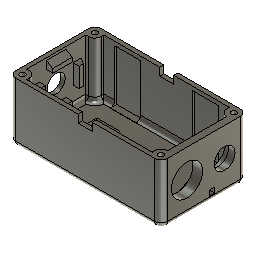
SolderungStationV2_Case_ESD_v2.8 (Autodesk Fusion 360 design; units mm, degrees)
Autodesk Fusion 360 part; units mm, degrees
sketch "草图1" plane through (0, 0, 0) normal (0, 0, 1) x (1, 0, 0)
  line L0 (2.5, 0) -> (56, 0)
  line L1 (58.5, -2.5) -> (58.5, -30.5)
  line L2 (56, -33) -> (2.5, -33)
  line L3 (0, -30.5) -> (0, -2.5)
  line L4 (0, -27.9) -> (2.6, -27.9)
  line L5 (5.1, -30.4) -> (5.1, -33)
  line L6 (58.5, -27.9) -> (55.9, -27.9)
  line L7 (53.4, -30.4) -> (53.4, -33)
  line L8 (53.4, 0) -> (53.4, -2.6)
  line L9 (55.9, -5.1) -> (58.5, -5.1)
  line L10 (5.1, 0) -> (5.1, -2.6)
  line L11 (2.6, -5.1) -> (0, -5.1)
  circle A0 centre (2.535, -2.53) radius 1
  line L12 (2.535, -2.53) -> (55.965, -2.53) construction
  line L13 (55.965, -2.53) -> (55.965, -30.47) construction
  line L14 (55.965, -30.47) -> (2.535, -30.47) construction
  line L15 (2.535, -30.47) -> (2.535, -2.53) construction
  circle A1 centre (55.965, -2.53) radius 1
  circle A2 centre (55.965, -30.47) radius 1
  circle A3 centre (2.535, -30.47) radius 1
  line L16 (2.535, -30.47) -> (0, -33) construction
  line L17 (55.965, -30.47) -> (58.5, -33) construction
  line L18 (58.5, 0) -> (55.965, -2.53) construction
  line L19 (0, 0) -> (2.535, -2.53) construction
  arc A4 (2.5, 0) -> (0, -2.5) centre (2.5, -2.5) ccw
  arc A5 (58.5, -2.5) -> (56, 0) centre (56, -2.5) ccw
  arc A6 (56, -33) -> (58.5, -30.5) centre (56, -30.5) ccw
  arc A7 (0, -30.5) -> (2.5, -33) centre (2.5, -30.5) ccw
  arc A8 (2.6, -5.1) -> (5.1, -2.6) centre (2.6, -2.6) ccw
  arc A9 (5.1, -30.4) -> (2.6, -27.9) centre (2.6, -30.4) ccw
  arc A10 (53.4, -2.6) -> (55.9, -5.1) centre (55.9, -2.6) ccw
  arc A11 (55.9, -27.9) -> (53.4, -30.4) centre (55.9, -30.4) ccw
  line L20 (56, -31.4) -> (2.5, -31.4)
  arc A12 (1.6, -30.5) -> (2.5, -31.4) centre (2.5, -30.5) ccw
  line L21 (1.6, -30.5) -> (1.6, -2.5)
  arc A13 (2.5, -1.6) -> (1.6, -2.5) centre (2.5, -2.5) ccw
  line L22 (2.5, -1.6) -> (56, -1.6)
  arc A14 (56.9, -2.5) -> (56, -1.6) centre (56, -2.5) ccw
  line L23 (56.9, -2.5) -> (56.9, -30.5)
  arc A15 (56, -31.4) -> (56.9, -30.5) centre (56, -30.5) ccw
  line L24 (55.96, -31.4) -> (55.96, -1.5)
  line L25 (10, -9.25) -> (18.9, -9.25)
  line L26 (18.9, -9.25) -> (18.9, -23.75)
  line L27 (18.9, -23.75) -> (10, -23.75)
  line L28 (10, -23.75) -> (10, -9.25)
  line L29 (0, -16.5) -> (58.5, -16.5)
  point P0 (5.1, -27.9)
  dimension "d1" = 58.5
  dimension "d2" = 33
  dimension "d5" = 1.6
  dimension "d6" = 5.1
  dimension "d7" = 2
  dimension "d10" = 53.43
  dimension "d11" = 27.94
  dimension "d12" = 2.5
  dimension "d28" = 2.5
  dimension "d37" = 2.54
  dimension "d75" = 14.5
  dimension "d77" = 8.9
  dimension "d78" = 10
  constraint horizontal L0
  constraint vertical L1
  constraint horizontal L2
  constraint vertical L3
  constraint coincident L19.start origin
  constraint coincident L3 L4.start
  constraint coincident L2 L5.end
  constraint perpendicular L2 L5
  constraint coincident L1 L6.start
  constraint perpendicular L1 L6
  constraint coincident L2 L7.end
  constraint perpendicular L2 L7
  constraint coincident L0 L8.start
  constraint perpendicular L0 L8
  constraint coincident L1 L9.end
  constraint perpendicular L1 L9
  constraint coincident L0 L10.start
  constraint perpendicular L10 L22
  constraint coincident L3 L11.end
  constraint perpendicular L3 L11
  constraint collinear L5 L10
  constraint collinear L4 L6
  constraint collinear L9 L11
  constraint horizontal L12
  constraint vertical L13
  constraint horizontal L14
  constraint vertical L15
  constraint coincident L12.end L13.start
  constraint coincident L13.end L14.start
  constraint coincident L14.end L15.start
  constraint coincident A0.centre L12.start
  constraint equal A0 A1
  constraint equal A0 A3
  constraint equal A0 A2
  constraint equal L16 L17
  constraint equal L17 L18
  constraint coincident L19.start L0
  constraint coincident L19.start L3
  constraint tangent L0 A4
  constraint tangent L3 A4
  constraint coincident L18.start L0
  constraint coincident L18.start L1
  constraint tangent L0 A5
  constraint tangent L1 A5
  constraint equal A4 A5
  constraint coincident L17.end L1
  constraint coincident L17.end L2
  constraint tangent L1 A6
  constraint tangent L2 A6
  constraint equal A4 A6
  constraint coincident L16.end L2
  constraint coincident L16.end L3
  constraint tangent L2 A7
  constraint tangent L3 A7
  constraint equal A4 A7
  constraint tangent L10 A8
  constraint tangent L11 A8
  constraint coincident P0 L5
  constraint coincident P0 L4
  constraint tangent L5 A9
  constraint tangent L4 A9
  constraint tangent L9 A10
  constraint tangent L8 A10
  constraint tangent L6 A11
  constraint tangent L7 A11
  constraint equal A9 A11
  constraint equal A8 A9
  constraint equal L4 L5
  constraint collinear L7 L8
  constraint equal A9 A10
  constraint equal L8 L9
  constraint equal L10 L11
  constraint coincident L20 L24.start
  constraint perpendicular L12 L24
  constraint horizontal L25
  constraint vertical L26
  constraint horizontal L27
  constraint vertical L28
  constraint midpoint L3 L29.start
  constraint midpoint L1 L29.end
  constraint symmetric L25 L27 L29
  measures "d1" distance of L19.start L18.start
  measures "d2" distance of L18.start L17.end
  measures "d6" distance of P0 L5.end
  measures "d7" diameter of A0
  measures "d10" distance of A0.centre L12.end
  measures "d11" distance of A0.centre L14.end
  measures "d12" radius of A4
  measures "d28" radius of A9
  measures "d37" distance of L1 L24
  measures "d75" distance of L25.end L26.end
  measures "d77" distance of L25.start L25.end
  measures "d78" distance of L3 L28
extrude "拉伸2" add sketch "草图1" along normal blind 1.6 contours L0 L3 L10 L11 A0 A4 L21 L22 | L0 L8 L10 L22 | L0 L1 L8 L9 A1 A5 L22 L23 | L8 L9 L10 L11 A8 A10 L21 L22 L24 L25 L26 L28 L29 | L10 L11 A0 A8 L21 L22 | L3 L11 L21 L29 | L8 L9 A1 A10 L22 L24 | A0 L21 A13 L22 | A0 L21 A13 L22 | L3 L4 L21 L29 | A1 L22 L24 | A1 L22 L24 | L2 L3 L4 L5 A3 A7 L20 L21 | L4 L5 L6 L7 A9 A11 L20 L21 L24 L26 L27 L28 L29 | L1 L9 L23 L29 | A1 L22 A14 L23 L24 | A1 L22 A14 L23 L24 | L9 A1 L23 L24 | L4 L5 A3 A9 L20 L21 | L1 L6 L23 L29 | L9 L23 L24 L29 | A3 L20 A12 L21 | A3 L20 A12 L21 | L1 L2 L6 L7 A2 A6 L20 L23 | L6 L23 L24 L29 | L2 L5 L7 L20 | L6 A2 L23 L24 | L6 L7 A2 A11 L20 L24 | A2 L20 L23 A15 L24 | A2 L20 L23 A15 | A2 L20 L24 makes body 1
extrude "拉伸3" add sketch "草图1" along normal blind 23 separate body contours L0 L3 L10 L11 A0 A4 L21 L22 | L0 L8 L10 L22 | L0 L1 L8 L9 A1 A5 L22 L23 | L10 L11 A0 A8 L21 L22 | L3 L11 L21 L29 | L8 L9 A1 A10 L22 L24 | A0 L21 A13 L22 | A0 L21 A13 L22 | L3 L4 L21 L29 | A1 L22 L24 | A1 L22 L24 | L2 L3 L4 L5 A3 A7 L20 L21 | L1 L9 L23 L29 | A1 L22 A14 L23 L24 | A1 L22 A14 L23 L24 | L9 A1 L23 L24 | L4 L5 A3 A9 L20 L21 | L1 L6 L23 L29 | L9 L23 L24 L29 | A3 L20 A12 L21 | A3 L20 A12 L21 | L1 L2 L6 L7 A2 A6 L20 L23 | L6 L23 L24 L29 | L2 L5 L7 L20 | L6 A2 L23 L24 | L6 L7 A2 A11 L20 L24 | A2 L20 L23 A15 L24 | A2 L20 L23 A15 | A2 L20 L24 makes body 2
combine "合并1" operation add target body 2 tool bodies 1
sketch "草图3" plane through (55.96, 0, 0) normal (-1, 0, 0) x (0, 1, 0)
  circle A0 centre (-23, -12) radius 6
  circle A1 centre (-8.5, -12) radius 4
  line L0 (-23, -12) -> (-8.5, -12) construction
  line L1 (-16.5, -1.6) -> (-16.5, -23) construction
  line L2 (-30.5, -16.3301) -> (-23, -20.6603)
  line L3 (-23, -20.6603) -> (-15.5, -16.3301)
  line L4 (-15.5, -16.3301) -> (-15.5, -7.6699)
  line L5 (-15.5, -7.6699) -> (-23, -3.3397)
  line L6 (-23, -3.3397) -> (-30.5, -7.6699)
  line L7 (-30.5, -7.6699) -> (-30.5, -16.3301)
  line L8 (-5.1, -1.6) -> (-27.9, -1.6)
  line L9 (-27.9, -1.6) -> (-27.9, -23)
  line L10 (-27.9, -23) -> (-5.1, -23)
  line L11 (-5.1, -23) -> (-5.1, -1.6)
  line L12 (-1, -12) -> (-32, -12)
  line L13 (-32, -12) -> (-32, -0.6011)
  line L14 (-32, -0.6011) -> (-1, -0.6011)
  line L15 (-1, -0.6011) -> (-1, -12)
  line L16 (-15.5, -16.3301) -> (-13.1332, -14.9637)
  line L17 (-13.5746, -14.121) -> (-13.5746, -15.2185)
  circle A2 centre (-8.5, -12) radius 5.5
  line L18 (-14.4011, -4.3276) -> (-12.4011, -4.3276)
  line L19 (-12.4011, -4.3276) -> (-12.4011, -2.3276)
  line L20 (-12.4011, -2.3276) -> (-14.4011, -2.3276)
  line L21 (-14.4011, -2.3276) -> (-14.4011, -4.3276)
  point P0 (-23, -12)
  point P1 (-8.5, -12)
  dimension "d31" = 12
  dimension "d32" = 8
  dimension "d34" = 6.5
  dimension "d35" = 8
  dimension "d38" = 7.5
  dimension "d39" = 11
  dimension "d51" = 11
  dimension "d99" = 2
  constraint coincident P0 A0.centre
  constraint coincident P1 A1.centre
  constraint horizontal L0
  constraint vertical L1
  constraint midpoint L1.end L10
  constraint midpoint L1.start L8
  constraint vertical L7
  constraint horizontal L12
  constraint vertical L13
  constraint horizontal L14
  constraint vertical L15
  constraint collinear L3 L16
  constraint coincident L16 L17.end
  constraint concentric A1 A2
  constraint coincident L16.end A2
  constraint collinear L0 L12
  constraint coincident L17.start A2
  constraint vertical L17
  constraint horizontal L18
  constraint vertical L19
  constraint horizontal L20
  constraint vertical L21
  constraint equal L18 L19
  measures "d31" diameter of A0
  measures "d32" diameter of A1
  measures "d34" distance of P0 L1
  measures "d35" distance of P1 L1
  measures "d38" distance of P0 L7
  measures "d39" distance of L0 L10
  measures "d51" diameter of A2
  measures "d99" distance of L18.start L18.end
extrude "拉伸7" add sketch "草图3" along normal blind 2.56 contours L4 L12 L16 L17 A2 | L4 L5 L6 L8 L9 L11 L12 A2 | L6 L7 L8 L9 L11 L12 L13 L14 L15 A2 | L18 L19 L20 L21 bodies 2
extrude "拉伸5" cut sketch "草图3" along normal blind 10 contours A0 L9 L12 | A0 L2 L3 L4 L9 L12 | A0 L4 L5 L6 L9 L12 | A0 L9 L12 | A0 L9 L12 | A0 L6 L7 L9 L12 | A0 L2 L7 L9 L12 | A0 L9 L12 | A1 L11 L12 A2 | A1 L11 L12 A2 | A1 L11 L12 | A1 L11 L12 | A1 L11 L12 A2 | A1 L11 L12 | A1 L11 L12 | A1 L11 L12 A2 bodies 2
extrude "拉伸8" add sketch "草图3" along normal blind 1.2 contours A0 L9 L12 | A0 L2 L3 L4 L9 L12 | A0 L4 L5 L6 L9 L12 | A0 L9 L12 | A0 L9 L12 | A0 L6 L7 L9 L12 | A0 L2 L7 L9 L12 | A0 L9 L12 bodies 2
extrude "拉伸4" cut sketch "草图3" along normal mid plane 10 contours A0 L9 L12 | A0 L9 L12 | A0 L9 L12 | A0 L9 L12 | A1 L11 L12 | A1 L11 L12 | A1 L11 L12 | A1 L11 L12 | L18 L19 L20 L21 bodies 2
sketch "草图2" plane through (0, 0, 23) normal (0, 0, 1) x (-1, 0, 0)
  line L0 (-5.1, 1.6) -> (-53.4, 1.6)
  line L1 (-53.4, 31.4) -> (-5.1, 31.4)
  line L2 (-1.6, 27.9) -> (-1.6, 5.1)
  arc A0 (-2.5, 0) -> (0, 2.5) centre (-2.5, 2.5) ccw
  line L3 (0, 2.5) -> (0, 30.5)
  arc A1 (0, 30.5) -> (-2.5, 33) centre (-2.5, 30.5) ccw
  line L4 (-2.5, 33) -> (-56, 33)
  arc A2 (-56, 33) -> (-58.5, 30.5) centre (-56, 30.5) ccw
  line L5 (-58.5, 30.5) -> (-58.5, 2.5)
  arc A3 (-58.5, 2.5) -> (-56, 0) centre (-56, 2.5) ccw
  line L6 (-56, 0) -> (-2.5, 0)
  circle A4 centre (-2.535, 30.47) radius 1
  circle A5 centre (-2.535, 2.53) radius 1
  circle A6 centre (-55.965, 2.53) radius 1
  circle A7 centre (-55.965, 30.47) radius 1
  line L7 (-5.1, 2.6) -> (-5.1, 1.6)
  line L8 (-53.4, 30.4) -> (-53.4, 31.4)
  arc A8 (-53.4, 2.6) -> (-55.9, 5.1) centre (-55.9, 2.6) ccw
  line L9 (-55.9, 5.1) -> (-55.96, 5.1)
  line L10 (-55.96, 27.9) -> (-55.9, 27.9)
  arc A9 (-55.9, 27.9) -> (-53.4, 30.4) centre (-55.9, 30.4) ccw
  line L11 (-5.1, 31.4) -> (-5.1, 30.4)
  arc A10 (-5.1, 30.4) -> (-2.6, 27.9) centre (-2.6, 30.4) ccw
  line L12 (-2.6, 27.9) -> (-1.6, 27.9)
  line L13 (-1.6, 5.1) -> (-2.6, 5.1)
  arc A11 (-2.6, 5.1) -> (-5.1, 2.6) centre (-2.6, 2.6) ccw
  line L14 (-53.4, 1.6) -> (-53.4, 2.6)
  line L15 (-55.96, 5.1) -> (-55.96, 27.9)
hole "孔1" at (2.535, -30.47, 23) at (2.535, -2.53, 23) at (56, -30.5, 23) at (56, -2.5, 23) direction (0, 0, -1) diameter 2 depth 8 tip angle 180 bodies 2
sketch "草图4" plane through (0, 0, 0) normal (0, 1, 0) x (1, 0, 0)
  line L0 (2.5, 0) -> (2.5, -23)
  line L1 (2.5, -23) -> (56, -23)
  line L2 (56, -23) -> (56, 0)
  line L3 (56, 0) -> (2.5, 0)
  line L4 (0, 0) -> (0, -23)
  line L5 (0, -23) -> (2.5, -23)
  line L6 (2.5, -23) -> (2.5, 0)
  line L7 (0, 0) -> (2.5, 0)
  line L8 (56, 0) -> (56, -23)
  line L9 (56, -23) -> (58.5, -23)
  line L10 (58.5, -23) -> (58.5, 0)
  line L11 (56, 0) -> (58.5, 0)
  line L12 (29.25, -23) -> (29.25, 0)
  line L13 (36.5, -23) -> (22, -23)
  line L14 (22, -23) -> (22, -11.1)
  line L15 (22, -11.1) -> (36.5, -11.1)
  line L16 (36.5, -11.1) -> (36.5, -23)
  line L17 (36.5, -20) -> (22, -20)
  line L18 (26.55, -23) -> (26.55, -20)
  line L19 (31.95, -20) -> (31.95, -23)
  dimension "d57" = 14.5
  dimension "d59" = 8.9
  dimension "d60" = 3
  dimension "d65" = 5.4
  constraint midpoint L1 L12.start
  constraint midpoint L3 L12.end
  constraint horizontal L13
  constraint vertical L14
  constraint horizontal L15
  constraint vertical L16
  constraint collinear L1 L13
  constraint coincident L16 L17.start
  constraint coincident L14 L17.end
  constraint perpendicular L14 L17
  constraint coincident L1 L18.start
  constraint coincident L13 L18.start
  constraint coincident L17 L18.end
  constraint perpendicular L17 L18
  constraint coincident L17 L19.start
  constraint coincident L1 L19.end
  constraint perpendicular L17 L19
  constraint symmetric L12 L18 L19
  constraint symmetric L12 L14 L16
  measures "d57" distance of L13.start L13.end
  measures "d59" distance of L14.end L17.end
  measures "d60" distance of L13.end L17.end
  measures "d65" distance of L18 L19
extrude "拉伸10" cut sketch "草图4" against normal blind 35 contours L1 L12 L13 L17 L18 | L1 L12 L13 L17 L19 bodies 2
sketch "草图5" plane through (0, 0, 0) normal (-1, 0, 0) x (0, -1, 0)
  line L0 (30.5, 0) -> (30.5, 23)
  line L1 (30.5, 23) -> (2.5, 23)
  line L2 (2.5, 23) -> (2.5, 0)
  line L3 (2.5, 0) -> (30.5, 0)
  circle A0 centre (16.5, 12.5) radius 3.45
  circle A1 centre (16.5, 12.5) radius 7.5 construction
  line L4 (23, 19) -> (10, 19)
  line L5 (10, 19) -> (10, 6)
  line L6 (10, 6) -> (23, 6)
  line L7 (23, 6) -> (23, 19)
  line L8 (24.6, 20.6) -> (8.4, 20.6)
  line L9 (8.4, 20.6) -> (8.4, 4.4)
  line L10 (8.4, 4.4) -> (24.6, 4.4)
  line L11 (24.6, 4.4) -> (24.6, 20.6)
  line L12 (12.7583, 19) -> (12.7583, 20.6)
  line L13 (20.2417, 19) -> (20.2417, 20.6)
  line L14 (10, 16.2417) -> (8.4, 16.2417)
  line L15 (23, 16.2417) -> (24.6, 16.2417)
  line L16 (10, 8.7583) -> (8.4, 8.7583)
  line L17 (12.7583, 6) -> (12.7583, 4.4)
  line L18 (20.2417, 6) -> (20.2417, 4.4)
  line L19 (23, 8.7583) -> (24.6, 8.7583)
  line L20 (16.5, 23) -> (16.5, 0)
  point P0 (16.5, 12.5)
  dimension "d66" = 6.9
  dimension "d67" = 15
  dimension "d68" = 6.5
  dimension "d69" = 1.6
  dimension "d74" = 10.5
  constraint concentric A0 A1
  constraint coincident P0 A0.centre
  constraint coincident A1 L12.start
  constraint coincident L4 L12.start
  constraint coincident L8 L12.end
  constraint perpendicular L8 L12
  constraint coincident L4 L13.start
  constraint coincident A1 L13.start
  constraint coincident L8 L13.end
  constraint perpendicular L8 L13
  constraint coincident L5 L14.start
  constraint coincident A1 L14.start
  constraint coincident L9 L14.end
  constraint perpendicular L9 L14
  constraint coincident A1 L15.start
  constraint coincident L7 L15.start
  constraint coincident L11 L15.end
  constraint perpendicular L11 L15
  constraint coincident L5 L16.start
  constraint coincident A1 L16.start
  constraint coincident L9 L16.end
  constraint perpendicular L9 L16
  constraint coincident L6 L17.start
  constraint coincident A1 L17.start
  constraint coincident L10 L17.end
  constraint perpendicular L10 L17
  constraint coincident A1 L18.start
  constraint coincident L6 L18.start
  constraint coincident L10 L18.end
  constraint perpendicular L10 L18
  constraint coincident A1 L19.start
  constraint coincident L7 L19.start
  constraint coincident L11 L19.end
  constraint perpendicular L11 L19
  constraint midpoint L1 L20.start
  constraint midpoint L3 L20.end
  constraint coincident P0 L20
  constraint vertical L7
  measures "d66" diameter of A0
  measures "d67" diameter of A1
  measures "d68" distance of P0 L7
  measures "d74" distance of P0 L20.start
extrude "拉伸11" add sketch "草图5" against normal blind 4 contours L6 L10 L18 L20 | L6 L10 L17 L20 | L4 L8 L12 L20 | L4 L8 L13 L20 | L5 L9 L14 L16 | L7 L11 L15 L19 bodies 2
extrude "拉伸12" cut sketch "草图5" against normal blind 8 contours A0 L20 | A0 L20 bodies 2
ref_plane "工作平面3" through (29.25, -0.8, 11.5) normal (0, 1, 0) x (-1, 0, 0)
sketch "草图6" plane through (29.25, -0.8, 11.5) normal (0, 1, 0) x (1, 0, 0)
  line L0 (-20, -10) -> (-10, -10)
  line L1 (-10, -10) -> (-10, 10)
  line L2 (-10, 10) -> (-20, 10)
  line L3 (-20, 10) -> (-20, -10)
  line L4 (2.7, -8.5) -> (2.7, -11.5)
  line L5 (2.7, -11.5) -> (26.75, -11.5)
  line L6 (26.75, -11.5) -> (26.75, 11.5)
  line L7 (26.75, 11.5) -> (-26.75, 11.5)
  line L8 (-26.75, 11.5) -> (-26.75, -11.5)
  line L9 (-26.75, -11.5) -> (-2.7, -11.5)
  line L10 (-2.7, -11.5) -> (-2.7, -8.5)
  line L11 (-2.7, -8.5) -> (2.7, -8.5)
  line L12 (-29.25, 11.5) -> (-29.25, -11.5)
  line L13 (-29.25, -11.5) -> (-26.75, -11.5)
  line L14 (-26.75, -11.5) -> (-26.75, 11.5)
  line L15 (-29.25, 11.5) -> (-26.75, 11.5)
  line L16 (26.75, 11.5) -> (26.75, -11.5)
  line L17 (26.75, -11.5) -> (29.25, -11.5)
  line L18 (29.25, -11.5) -> (29.25, 11.5)
  line L19 (26.75, 11.5) -> (29.25, 11.5)
  line L20 (-29.25, 0) -> (29.25, 0)
  line L21 (0, -19) -> (0, 17)
  line L22 (20, 10) -> (20, -10)
  line L23 (20, -10) -> (10, -10)
  line L24 (10, 10) -> (20, 10)
  line L25 (10, -10) -> (10, 10)
  dimension "d79" = 10
  dimension "d80" = 20
  dimension "d84" = 10
  constraint horizontal L0
  constraint vertical L1
  constraint horizontal L2
  constraint vertical L3
  constraint midpoint L12 L20.start
  constraint midpoint L18 L20.end
  constraint symmetric L0 L2 L20
  constraint perpendicular L20 L21
  constraint symmetric L0.start L21 L22.end
  constraint symmetric L0.end L21 L23.end
  constraint symmetric L1.end L21 L24.start
  constraint symmetric L2.end L21 L22.start
  measures "d79" distance of L0.start L0.end
  measures "d80" distance of L0.start L2.end
  measures "d84" distance of origin L1
extrude "拉伸13" cut sketch "草图6" against normal blind 2.5 contours L0 L1 L3 L20 | L1 L2 L3 L20 | L20 L22 L24 L25 | L20 L22 L23 L25 bodies 2
ref_plane "工作平面4" through (29.25, -32.2, 11.5) normal (0, -1, 0) x (1, 0, 0)
sketch "草图7" plane through (29.25, -32.2, 11.5) normal (0, -1, 0) x (1, 0, 0)
  line L0 (-20, -10) -> (-20, 10)
  line L1 (-20, 10) -> (-10, 10)
  line L2 (-10, 10) -> (-10, -10)
  line L3 (-10, -10) -> (-20, -10)
  line L4 (20, -10) -> (20, 10)
  line L5 (20, 10) -> (10, 10)
  line L6 (10, 10) -> (10, -10)
  line L7 (10, -10) -> (20, -10)
extrude "拉伸14" cut sketch "草图7" against normal blind 2.5 bodies 2
fillet "圆角1" radius 2 8 edges at (57.7678, -32.2678, 0) (29.25, -33, 0) (0.7322, -32.2678, 0) (0, -16.5, 0) (0.7322, -0.7322, 0) (29.25, 0, 0) (57.7678, -0.7322, 0) (58.5, -16.5, 0) on bodies 2
chamfer "倒角1" distance 1.5 distance2 2.4 4 edges at (1.6, -16.5, 20.6) (1.6, -24.6, 12.5) (1.6, -8.4, 12.5) (1.6, -16.5, 4.4) measured on face at (1.6, -24.2472, 4.9194) measured on face at (1.6, -24.2472, 4.9194) measured on face at (1.6, -24.2472, 4.9194) measured on face at (1.6, -24.2472, 4.9194) on bodies 2
fillet "圆角2" radius 1.7 14 edges at (29.25, -1.6, 1.6) (51.325, -1.6, 1.6) (53.4, -16.5, 1.6) (51.325, -31.4, 1.6) (29.25, -31.4, 1.6) (7.175, -31.4, 1.6) (5.1, -30.9, 1.6) (4.3678, -28.6322, 1.6) (2.1, -27.9, 1.6) (1.6, -16.5, 1.6) (2.1, -5.1, 1.6) (4.3678, -4.3678, 1.6) (5.1, -2.1, 1.6) (7.175, -1.6, 1.6) on bodies 2
named bodies: "实体1", "Box"
